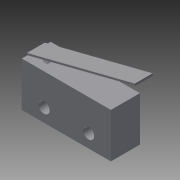
# Autodesk Inventor part: lever switch 20x10x6
Saved by Autodesk Inventor 2013 SP2 (Build 170200200, 200)
## iProperties
Created: 2017-05-25
Part Number: lever switch 20x10x6
Material: Generic
Document SubType Name: Modeling
Designer: Herman de Vries
Density: 1 g/cm^3
Author: Herman de Vries
Autodesk Inventor part; units mm, degrees
ref_plane "YZ Plane" through (0, 0, 0) normal (1, 0, 0) x (0, 1, 0)
ref_plane "XZ Plane" through (0, 0, 0) normal (0, 1, 0) x (-1, 0, 0)
sketch "Sketch1" plane through (0, 0, 0) normal (0, 0, 1) x (1, 0, 0)
  line L0 (0, 0) -> (20, 0)
  line L1 (20, 0) -> (20, 6.5)
  line L2 (20, 6.5) -> (0, 6.5)
  line L3 (0, 6.5) -> (0, 0)
  dimension "d0" = 20
  dimension "d1" = 6.5
  constraints: 8 end point, 2 parallel, 1 horizontal, 1 perpendicular
  measures "d0" distance of L2.end L1.end
  measures "d1" distance of L1.end L0.end
extrude "Extrusion1" add sketch "Sketch1" along normal blind 10
sketch "Sketch2" plane through (0, 0, 10) normal (0, 0, 1) x (1, 0, 0)
  line L0 (3, 4.75) -> (4, 4.75)
  line L1 (4, 4.75) -> (4, 1.75)
  line L2 (4, 1.75) -> (3, 1.75)
  line L3 (3, 1.75) -> (3, 4.75)
  line L4 (0, 6.5) -> (0, 0) projected
  point P0 (3, 3.25)
  point P1 (0, 3.25)
  dimension "d4" = 1
  dimension "d5" = 3
  dimension "d6" = 3
  constraints: 8 end point, 2 midpoint, 2 parallel, 1 horizontal, 1 horizontal alignment, 1 perpendicular
  measures "d4" distance of L1.end L2.end
  measures "d5" distance of L0.end L1.end
  measures "d6" distance between parallel lines of L4 L3
extrude "Extrusion2" add sketch "Sketch2" along normal blind 1
sketch "Sketch3" plane through (0, 0, 0) normal (0, -1, 0) x (1, 0, 0)
  circle A0 centre (5, 3) radius 1.25
  circle A1 centre (15, 3) radius 1.25
  line L0 (5, 3) -> (15, 3) construction
  line L1 (0, 0) -> (20, 0) construction
  point P0 (10, 3)
  point P1 (10, 0)
  dimension "d9" = 2.5
  dimension "d10" = 2.5
  dimension "d11" = 3
  dimension "d12" = 10
  constraints: 2 centre point, 2 end point, 2 midpoint, 1 horizontal, 1 horizontal alignment, 1 vertical alignment
  measures "d9" diameter of A0
  measures "d10" diameter of A1
  measures "d11" distance between parallel lines of L1 L0
  measures "d12" distance of L0.start L0.end
extrude "Extrusion3" cut sketch "Sketch3" against normal through all
ref_plane "Work Plane1" through (0, 3.25, 0) normal (0, -1, 0) x (1, 0, 0)
sketch "Sketch4" plane through (0, 3.25, 0) normal (0, -1, 0) x (1, 0, 0)
  line L0 (0, 10) -> (-0.1016, 10.4)
  line L1 (-0.1016, 10.4) -> (24.1283, 16.5571)
  line L2 (24.1283, 16.5571) -> (24.2299, 16.1571)
  line L3 (24.2299, 16.1571) -> (0, 10)
  dimension "d15" = 0.4
  dimension "d19" = 25
  constraints: 8 end point, 2 parallel, 1 coincident, 1 perpendicular
  measures "d15" vertical distance of L0.start L0.end
  measures "d19" distance of L0.end L1.end
extrude "Extrusion4" add sketch "Sketch4" along normal mid plane 4
body "Solid1"
